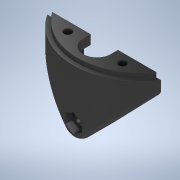
# Autodesk Inventor part: WheelBracketHead
Saved by Autodesk Inventor 2020 (Build 240168000, 168)
## iProperties
Created: 2019-05-28
Part Number: WheelBracketHead
Material: ABS Plastic
Document SubType Name: Modeling
Designer: Connor
Density: 1.06 g/cm^3
Appearance: Glossy - Black
Author: Connor
Autodesk Inventor part; units mm, degrees
ref_plane "YZ Plane" through (0, 0, 0) normal (1, 0, 0) x (0, 1, 0)
sketch "Sketch1" plane through (0, 0, 0) normal (0, 0, 1) x (1, 0, 0)
  line L0 (0, 0) -> (46.99, 0)
  line L1 (46.99, 0) -> (46.99, 44.45)
  line L2 (46.99, 44.45) -> (0, 44.45)
  line L3 (0, 44.45) -> (0, 0)
  line L4 (0, 44.45) -> (44.196, 44.45)
  line L5 (44.196, 44.45) -> (44.196, 47.6504)
  line L6 (44.196, 47.6504) -> (0, 47.6504)
  line L7 (0, 47.6504) -> (0, 44.45)
  circle A0 centre (0, 9.525) radius 9.525
  circle A1 centre (0, 9.525) radius 3.175
  line L8 (46.99, 44.45) -> (6.8499, 2.9065)
  line L9 (0, 0) -> (-46.99, 0)
  line L10 (-46.99, 0) -> (-46.99, 44.45)
  line L11 (-46.99, 44.45) -> (0, 44.45)
  line L12 (0, 44.45) -> (0, 0)
  line L13 (-46.99, 44.45) -> (-6.8499, 2.9065)
  dimension "d2" = 44.196
  dimension "d3" = 3.2004
  dimension "d5" = 6.35
  dimension "d7" = 6.35
  dimension "d67" = 34.925
  dimension "d119" = 46.99
  constraints: 28 end point, 6 parallel, 3 horizontal, 3 perpendicular, 3 point on circle, 2 centre point, 2 equal length, 2 tangent, 1 coincident, 1 point on line
  measures "d2" distance of L6.end L5.end
  measures "d3" distance of L5.end L4.end
  measures "d5" diameter of A1
  measures "d7" radial gap between concentric circles of A1 A0
  measures "d67" distance from line of L11 A0.centre
  measures "d119" distance between parallel lines of L7 L1
revolve "Revolution1" add sketch "Sketch1" angle 180 about axis through (0, 44.45, 0) along (0, -1, 0) picked at (7.3287, 10.2315) picked at (0.9535, 9.9842) contours A0 L8 L1 L0 | L3 A1 A0 | L3 A1 | A0 L3 L2 L8 | L2 L7 L6 L5
sketch "Sketch2" plane through (0, 0, 0) normal (1, 0, 0) x (0, 1, 0)
  line L0 (0, 0) -> (44.45, 0) projected
  line L1 (47.6504, 44.196) -> (47.6504, 0) projected
  line L2 (0, 0) -> (47.6504, 0)
  line L3 (47.6504, 0) -> (47.6504, 25.4)
  line L4 (47.6504, 25.4) -> (0, 25.4)
  line L5 (0, 25.4) -> (0, 0)
  point P0 (44.45, 0)
  dimension "d10" = 25.4
  constraints: 8 end point, 2 parallel, 1 horizontal, 1 perpendicular, 1 point on line
  measures "d10" distance between parallel lines of L0 L4
extrude "Extrusion1" cut sketch "Sketch2" along normal through all both and the other way through all
extrude "Extrusion2" cut sketch "Sketch1" along normal through all contours A0 L8 L1 L0 | L9 L10 L13 A0
ref_plane "Work Plane1" through (0, 0, 0) normal (0, 1, 0) x (-1, 0, 0)
sketch "Sketch9" plane through (0, 0, 0) normal (0, 1, 0) x (-1, 0, 0)
  line L0 (-19.05, 31.75) -> (0, 0) construction
  line L1 (0, 0) -> (19.05, 31.75) construction
  dimension "d46" = 31.75
  dimension "d47" = 38.1
  constraints: 4 end point, 1 equal length, 1 horizontal alignment
  measures "d46" vertical distance of L0.end L0.start
  measures "d47" distance of L1.end L0.start
hole "Hole1" at (19.05, 0, 31.75) at (-19.05, 0, 31.75) direction (0, 1, 0) diameter 5.207 end through all counterbore diameter 8.7313 counterbore depth 25.4
ref_plane "Work Plane2" through (0, 22.225, 46.99) normal (0, 0, 1) x (1, 0, 0)
sketch "Sketch10" plane through (0, 22.225, 46.99) normal (0, 0, 1) x (1, 0, 0)
  arc A0 (-6.8499, -19.3185) -> (6.8499, -19.3185) centre (0, -12.7) ccw projected
  point P0 (0, -22.225)
  point P1 (0, -12.7)
  constraints: 1 coincident
hole "Hole2" at (0, 9.525, 46.99) direction (0, 0, -1) diameter 6.7564 end through all
fillet "Fillet1" radius 0.7937 4 edges at (19.05, 15.5331, 36.1156) (-19.05, 15.5331, 36.1156) (-3.3781, 9.4995, 46.8684) (3.3781, 9.4966, 46.8684)
fillet "Fillet2" radius 3.175 4 edges at (3.9366, 0.8515, 46.8248) (-3.9366, 0.8515, 46.8248) (-25.4761, 22.1839, 39.4845) (25.4761, 22.1839, 39.4845)
sketch "Sketch12" plane through (0, 0, 0) normal (1, 0, 0) x (0, 1, 0)
  line L0 (12.9032, 25.4) -> (6.1468, 25.4) projected
  line L1 (41.3004, 20.955) -> (38.919, 16.1925)
  line L2 (30.3217, 16.1925) -> (22.225, 21.2094)
  line L3 (22.225, 21.2094) -> (22.225, 30.48)
  line L4 (47.6504, 30.48) -> (22.225, 30.48)
  line L5 (47.6504, 30.48) -> (47.6504, 20.955)
  line L6 (47.6504, 20.955) -> (41.3004, 20.955)
  line L7 (38.919, 16.1925) -> (30.3217, 16.1925)
  line L8 (47.6504, 44.196) -> (47.6504, 25.4) projected
  point P0 (0, 0)
  point P1 (9.525, 25.4)
  dimension "d102" = 14.2875
  dimension "d105" = 63.433
  dimension "d106" = 31.783
  dimension "d107" = 9.525
  dimension "d108" = 12.7
  dimension "d109" = 9.525
  dimension "d110" = 6.35
  dimension "d111" = 30.48
  constraints: 14 end point, 2 horizontal, 2 vertical, 1 collinear, 1 midpoint
  measures "d102" distance between parallel lines of L7 L4
  measures "d105" angle of L7 L1
  measures "d106" angle of L7 L2
  measures "d107" distance of L4.start L5.end
  measures "d108" distance from line of point (9.525, 25.4) L3
  measures "d109" distance of L2.start L2.end
  measures "d110" distance of L5.end L1.start
  measures "d111" distance from line of point (0, 0) L4
revolve "Revolution2" cut sketch "Sketch12" angle 360 about axis through (0, 47.6504, 30.48) along (0, -1, 0)
sketch "Sketch13" plane through (0, 22.225, 46.99) normal (0, 0, 1) x (1, 0, 0)
  circle A0 centre (0, -12.7) radius 3.3782 projected
  line L0 (0, -6.1375) -> (5.6832, -9.4188)
  line L1 (5.6832, -9.4188) -> (5.6832, -15.9812)
  line L2 (5.6832, -15.9812) -> (0, -19.2625)
  line L3 (0, -19.2625) -> (-5.6832, -15.9812)
  line L4 (-5.6832, -15.9812) -> (-5.6833, -9.4188)
  line L5 (-5.6833, -9.4188) -> (0, -6.1375)
  point P0 (0, -22.225)
  dimension "d91" = 11.3665
  constraints: 12 end point, 1 coincident, 1 vertical alignment, 13 other
  measures "d91" distance between parallel lines of L3 L0
extrude "Extrusion8" cut sketch "Sketch13" against normal blind 4.7625
sketch "Sketch14" plane through (39.5335, 44.45, 25.4) normal (0, 0, -1) x (-1, 0, 0)
  line L0 (30.2629, -22.225) -> (25.246, -14.1283) projected
  line L1 (48.8041, -22.225) -> (30.2629, -22.225) projected
  line L2 (48.8041, -22.225) -> (53.821, -14.1283) projected
  line L3 (53.821, -5.531) -> (49.0585, -3.1496) projected
  line L4 (25.246, -5.531) -> (30.0085, -3.1496) projected
  line L5 (30.0085, -3.1496) -> (30.0085, 3.2004) projected
  line L6 (49.0585, -3.1496) -> (49.0585, 3.2004) projected
  line L7 (30.0085, 3.2004) -> (49.0585, 3.2004) projected
  line L8 (49.0585, -3.1496) -> (30.0085, -3.1496) projected
  line L9 (25.246, -14.1283) -> (25.246, -5.531) projected
  line L10 (53.821, -14.1283) -> (53.821, -5.531) projected
  point P0 (39.5335, -44.45)
  point P1 (47.2884, -22.225)
  point P2 (31.7787, -22.225)
  point P3 (53.821, -5.531)
  point P4 (25.246, -5.531)
  point P5 (31.4763, 3.2004)
  point P6 (47.5908, 3.2004)
  point P7 (47.5908, -3.1496)
  point P8 (31.4763, -3.1496)
  constraints: 4 other
extrude "Extrusion9" cut sketch "Sketch14" against normal blind 5.08
sketch "Sketch15" plane through (0, 22.225, 30.48) normal (0, 1, 0) x (1, 0, 0)
  arc A0 (-9.525, 0) -> (9.525, 0) centre (0, 0) ccw projected
  circle A1 centre (0, 0) radius 6.477
  point P0 (0, 30.48)
  point P1 (7.9375, 0)
  point P2 (-7.9375, 0)
  point P3 (-5.715, -7.62)
  point P4 (5.715, -7.62)
  point P5 (-8.7938, 0)
  point P6 (8.7938, 0)
  dimension "d98" = 12.954
  constraints: 1 centre point, 1 coincident
  measures "d98" diameter of A1
hole "Hole5" at (0, 22.225, 30.48) direction (0, -1, 0) diameter 8.89 depth 6.35 counterbore diameter 12.954 counterbore depth 4.7752
body "Solid1"
